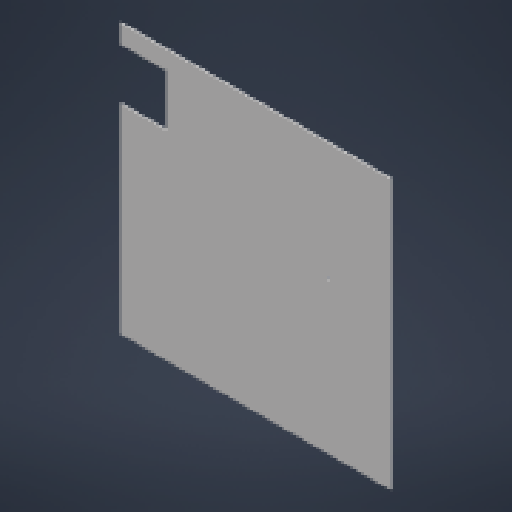
# Autodesk Inventor part: baseb
Saved by Autodesk Inventor 2026.2 (Build 302298000, 298)
## iProperties
Created: 2026-03-08
Part Number: baseb
Material: Generic
Document SubType Name: Modeling
Designer: danda
Density: 1 g/cm^3
Appearance: Default
Author: danda
Autodesk Inventor part; units mm, degrees
ref_plane "YZ Plane" through (0, 0, 0) normal (1, 0, 0) x (0, 1, 0)
ref_plane "XZ Plane" through (0, 0, 0) normal (0, 1, 0) x (-1, 0, 0)
ref_plane "XY Plane" through (0, 0, 0) normal (0, 0, 1) x (1, 0, 0)
sketch "Sketch1" plane through (0, 0, 0) normal (0, 0, 1) x (1, 0, 0)
  line L0 (4.7232, 12.5287) -> (1004.7232, 12.5287)
  line L1 (1004.7232, 12.5287) -> (1004.7232, -987.4713)
  line L2 (1004.7232, -987.4713) -> (4.7232, -987.4713)
  line L3 (4.7232, -987.4713) -> (4.7232, 12.5287)
  point P0 (0, 0)
  dimension "d0" = 1000
  dimension "d1" = 1000
  constraints: 8 end point, 2 parallel, 1 horizontal, 1 perpendicular
  measures "d0" distance of L1.end L2.end
  measures "d1" distance of L0.end L1.end
extrude "Extrusion1" add sketch "Sketch1" along normal blind 5
sketch "Sketch2" plane through (0, 0, 0) normal (0, 0, -1) x (-1, 0, 0)
  circle A0 centre (-775.6709, -419.8039) radius 6
  point P0 (0, 0)
  dimension "d4" = 12
  constraints: 1 centre point
  measures "d4" diameter of A0
extrude "Extrusion2" cut sketch "Sketch2" against normal blind 5
sketch "Sketch3" plane through (0, 0, 0) normal (0, 0, -1) x (-1, 0, 0)
  line L0 (-4.7232, 12.5287) -> (-4.7232, -987.4713) projected
  line L1 (-4.7232, -57.4713) -> (-174.7232, -57.4713)
  line L2 (-174.7232, -57.4713) -> (-174.7232, -247.4713)
  line L3 (-174.7232, -247.4713) -> (-4.7232, -247.4713)
  line L4 (-4.7232, -247.4713) -> (-4.7232, -57.4713)
  line L5 (-1004.7232, 12.5287) -> (-4.7232, 12.5287) projected
  point P0 (0, 0)
  dimension "d8" = 170
  dimension "d9" = 190
  dimension "d10" = 170
  dimension "d11" = 70
  constraints: 8 end point, 2 point on line, 1 collinear, 1 horizontal, 1 perpendicular
  measures "d8" distance of L1.start L1.end
  measures "d9" distance of L1.end L2.end
  measures "d10" distance of L2.end L3.end
  measures "d11" distance between parallel lines of L5 L1
extrude "Extrusion3" cut sketch "Sketch3" against normal through all
body "Solid1"
